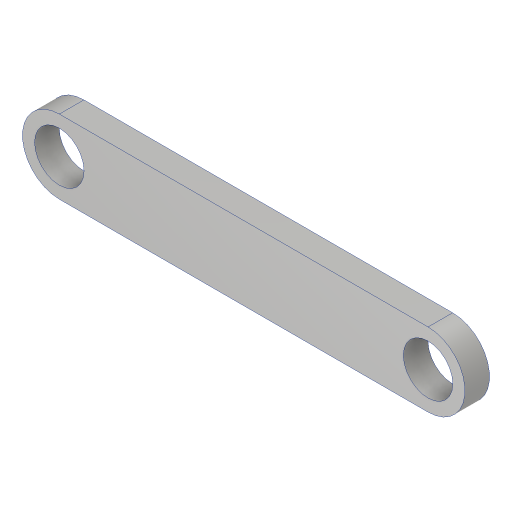
# Autodesk Inventor part: Link
Saved by Autodesk Inventor 2023.2 (Build 272271000, 271)
## iProperties
Created: 2021-07-28
Part Number: Link
Material: 알루미늄 6061
Document SubType Name: Modeling
Designer: user
Density: 2.7 g/cm^3
Appearance: 알루미늄 - 평지
Mass: 8.56168 g
Surface Area: 25.4742 cm^2
Volume: 3.17099 cm^3
Author: user
Autodesk Inventor part; units mm, degrees
ref_plane "YZ Plane" through (0, 0, 0) normal (1, 0, 0) x (0, 1, 0)
ref_plane "XZ Plane" through (0, 0, 0) normal (0, 1, 0) x (-1, 0, 0)
ref_plane "XY Plane" through (0, 0, 0) normal (0, 0, 1) x (1, 0, 0)
sketch "스케치1" plane through (0, 0, 0) normal (0, 0, 1) x (1, 0, 0)
  line L0 (0, 0) -> (-36, 0)
  line L1 (0, 0) -> (36, 0) construction
  line L2 (-36, 0) -> (-36, 6)
  line L3 (-36, 0) -> (-36, -6)
  line L4 (-36, 0) -> (-30, 0) construction
  line L5 (0, 0) -> (36, 0)
  line L6 (0, 0) -> (36, 0) construction
  line L7 (36, 0) -> (36, 6)
  line L8 (36, 0) -> (36, -6)
  line L9 (36, 0) -> (42, 0) construction
  line L10 (-36, -6) -> (36, -6)
  line L11 (-36, 6) -> (36, 6)
  circle A0 centre (-30, 0) radius 4.025
  circle A1 centre (30, 0) radius 4.025
  dimension "d0" = 36
  dimension "d1" = 180
  dimension "d2" = 6
  dimension "d3" = 90
  dimension "d4" = 6
  dimension "d5" = 90
  dimension "d6" = 0
  dimension "d7" = 36
  dimension "d8" = 6
  dimension "d9" = 6
  dimension "d10" = 90
  dimension "d11" = 8.05
  dimension "d12" = 8.05
  dimension "d13" = 6
  dimension "d14" = 6
  dimension "d15" = 30
  dimension "d16" = 30
  constraints: 24 end point, 5 horizontal, 4 equal length, 3 vertical, 2 centre point, 1 coincident, 1 perpendicular, 1 point on line
  measures "d0" distance of L0.start L0.end
  measures "d1" angle of L0 L1
  measures "d2" distance of L0.end L2.end
  measures "d3" angle of L0 L2
  measures "d4" distance of L0.end L3.end
  measures "d5" angle of L3 L4
  measures "d6" distance between parallel lines of L5 L6
  measures "d7" distance of L0.start L5.end
  measures "d8" distance of L6.end L7.end
  measures "d9" distance of L6.end L8.end
  measures "d10" angle of L8 L9
  measures "d11" diameter of A0
  measures "d12" diameter of A1
  measures "d13" distance from line of L3 L4.end
  measures "d14" distance from line of L8 A1.centre
  measures "d15" distance of L0.start L4.end
  measures "d16" distance of A1.centre L0.start
extrude "돌출1" add sketch "스케치1" along normal blind 4 contours L5 A1 L8 L10 L3 L0 A0 | L0 A0 L2 L11 L7 L5 A1
fillet "모깎기1" radius 6 2 edges at (36, -6, 2) (36, 6, 2)
fillet "모깎기2" radius 6 2 edges at (-36, -6, 2) (-36, 6, 2)
sketch "스케치4" plane through (0, 0, 0) normal (0, 0, -1) x (-1, 0, 0)
  circle A0 centre (30, 0) radius 4.025 projected
  circle A1 centre (30, 0) radius 4.8
  point P0 (0, 0)
  dimension "d27" = 9.6
  constraints: 1 centre point, 1 coincident
  measures "d27" diameter of A1
sketch "스케치5" plane through (0, 0, 0) normal (0, 0, -1) x (-1, 0, 0)
  circle A0 centre (30, 0) radius 4.8 projected
  arc A1 (30, -6) -> (30, 6) centre (30, 0) ccw projected
  line L0 (30, 6) -> (-30, 6) projected
  arc A2 (-30, 6) -> (-30, -6) centre (-30, 0) ccw projected
  line L1 (-30, -6) -> (30, -6) projected
  circle A3 centre (-30, 0) radius 4.035 projected
  circle A4 centre (-30, 0) radius 4.8
  point P0 (0, 0)
  constraints: 1 centre point, 1 coincident, 1 equal radius
